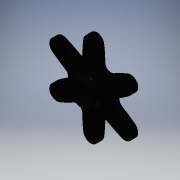
# Autodesk Inventor part: Sevo arm TowerPro SG-5010
Saved by Autodesk Inventor 2019 (Build 230136000, 136)
## iProperties
Created: 2015-05-13
Part Number: Sevo arm TowerPro SG-5010
Material: Ogólny
Document SubType Name: Modeling
Designer: Chaczyk
Density: 1 g/cm^3
Appearance: Domyślna
Author: Chaczyk
Autodesk Inventor part; units mm, degrees
ref_plane "YZ Plane" through (0, 0, 0) normal (1, 0, 0) x (0, 1, 0)
ref_plane "XZ Plane" through (0, 0, 0) normal (0, 1, 0) x (-1, 0, 0)
ref_plane "XY Plane" through (0, 0, 0) normal (0, 0, 1) x (1, 0, 0)
sketch "Szkic1" plane through (0, 0, 0) normal (0, 1, 0) x (-1, 0, 0)
  circle A0 centre (0, 0) radius 3.5
  line L0 (0, 0) -> (2.5, 0)
  line L1 (2.5, 0) -> (-2.5, 0)
  arc A1 (2.5, 13.012) -> (0, 15.5) centre (-0.142, 12.8573) ccw
  arc A2 (2.8239, 8.1091) -> (2.5, 13.012) centre (-52.6667, 6.905) ccw
  arc A3 (0, 15.5) -> (-2.5, 13.012) centre (0.142, 12.8573) ccw
  arc A4 (-2.5, 13.012) -> (-2.8239, 8.1091) centre (52.6667, 6.905) ccw
  circle A5 centre (0, 13.25) radius 0.5
  line L2 (3.8856, 6.386) -> (4.1618, 6.2393)
  arc A6 (2.8239, 8.1091) -> (3.8856, 6.386) centre (4.8235, 8.1525) ccw
  line L3 (-3.8856, 6.386) -> (-4.1618, 6.2393)
  arc A7 (-3.8856, 6.386) -> (-2.8239, 8.1091) centre (-4.8235, 8.1525) ccw
  line L4 (-4.1618, 6.2393) -> (4.1618, 6.2393)
  line L5 (0, 0) -> (0, 7.5)
  circle A8 centre (0, 7.5) radius 0.5
  line L6 (0, 13.25) -> (0, 7.5)
  circle A9 centre (0, 10.375) radius 0.5
  point P0 (2.837, 6.9427)
  point P1 (-2.837, 6.9427)
  dimension "d0" = 7
  dimension "d4" = 2.5
  dimension "d5" = 5
  dimension "d6" = 1
  dimension "d8" = 1.5
  dimension "d9" = 2
  dimension "d10" = 1.5
  dimension "d11" = 2
  dimension "d15" = 7.5
  dimension "d16" = 1
  dimension "d17" = 1
  constraints: 14 end point, 14 point on circle, 10 centre point, 4 tangent, 3 coincident, 3 point on line, 2 horizontal, 1 collinear, 1 midpoint, 1 vertical
  measures "d0" diameter of A0
  measures "d4" distance of L0.start L0.end
  measures "d5" distance of L0.end L1.end
  measures "d6" diameter of A5
  measures "d8" distance of point (2.837, 6.943) L2.end
  measures "d9" radius of A6
  measures "d10" distance of point (-2.837, 6.943) L3.end
  measures "d11" radius of A7
  measures "d15" distance of L0.start L5.end
  measures "d16" diameter of A8
  measures "d17" diameter of A9
sketch "Szkic2" plane through (0, 0, 0) normal (0, 1, 0) x (-1, 0, 0)
  circle A0 centre (0, 0) radius 7.5
  dimension "d12" = 15
  constraints: 1 centre point, 1 coincident
  measures "d12" diameter of A0
extrude "Wyciągnięcie proste1" add sketch "Szkic2" along normal blind 2
extrude "Wyciągnięcie proste2" add sketch "Szkic1" along normal blind 2 contours A2 A6 L2 L4 L3 A7 A4 A3 A1
pattern_circular "Szyk kołowy1" count 6 over 360 about axis through (0, 2, 0) along (0, 1, 0) of "Wyciągnięcie proste2"
sketch "Szkic3" plane through (0, 2, 0) normal (0, 1, 0) x (1, 0, 0)
  arc A0 (-0.4997, -7.4833) -> (0.4997, -7.4833) centre (0, 0) ccw projected
  circle A1 centre (0, -7.5) radius 0.5
  dimension "d23" = 1
  constraints: 1 centre point, 1 point on circle
  measures "d23" diameter of A1
extrude "Wyciągnięcie proste3" cut sketch "Szkic3" against normal blind 2
pattern_circular "Szyk kołowy2" count 6 over 360 about axis through (0, 2, 0) along (0, 1, 0) of "Wyciągnięcie proste3"
sketch "Szkic4" plane through (0, 2, 0) normal (0, 1, 0) x (1, 0, 0)
  circle A0 centre (0, 0) radius 3.5
  circle A1 centre (0, 0) radius 3.25
  dimension "d29" = 7
  dimension "d30" = 6.5
  constraints: 2 centre point, 2 coincident
  measures "d29" diameter of A0
  measures "d30" diameter of A1
extrude "Wyciągnięcie proste4" add sketch "Szkic4" along normal blind 0.5
sketch "Szkic5" plane through (0, 2, 0) normal (0, 1, 0) x (1, 0, 0)
  circle A0 centre (0, 0) radius 2
  dimension "d33" = 4
  constraints: 1 centre point, 1 coincident
  measures "d33" diameter of A0
extrude "Wyciągnięcie proste5" cut sketch "Szkic5" against normal blind 2
sketch "Szkic6" plane through (0, 0, 0) normal (0, -1, 0) x (1, 0, 0)
  circle A0 centre (0, 0) radius 4
  circle A1 centre (0, 0) radius 3.5
  dimension "d36" = 8
  dimension "d37" = 7
  constraints: 2 centre point, 2 coincident
  measures "d36" diameter of A0
  measures "d37" diameter of A1
extrude "Wyciągnięcie proste6" add sketch "Szkic6" along normal blind 3
fillet "Zaokrąglenie1" radius 2 1 edges at (-4, 0, 0)
fillet "Zaokrąglenie2" radius 0.25 1 edges at (-4, -3, 0)
fillet "Zaokrąglenie3" radius 0.25 1 edges at (-3.5, 2, 0)
sketch "Sketch7" plane through (0, 2, 0) normal (0, 1, 0) x (1, 0, 0)
  circle A0 centre (-6.4952, -3.75) radius 0.5 projected
  circle A1 centre (-6.4952, 3.75) radius 0.5 projected
  circle A2 centre (0, 7.5) radius 0.5 projected
  circle A3 centre (6.4952, 3.75) radius 0.5 projected
  circle A4 centre (6.4952, -3.75) radius 0.5 projected
  circle A5 centre (0, -7.5) radius 0.5 projected
  circle A6 centre (-11.4748, 6.625) radius 0.5 projected
  circle A7 centre (-8.985, 5.1875) radius 0.5 projected
  arc A8 (-5.6107, 6.5001) -> (-3.9339, 6.3855) centre (-4.6485, 8.2535) ccw projected
  arc A9 (-5.6107, 6.5001) -> (-10.0187, 8.6711) centre (-32.3132, -42.1582) ccw projected
  arc A10 (-10.0187, 8.6711) -> (-13.4234, 7.75) centre (-11.2058, 6.3057) ccw projected
  arc A11 (-13.4234, 7.75) -> (-12.5187, 4.3409) centre (-11.0638, 6.5516) ccw projected
  arc A12 (-12.5187, 4.3409) -> (-8.4346, 1.6089) centre (20.3535, 49.0631) ccw projected
  arc A13 (-7.4969, 0.2141) -> (-8.4346, 1.6089) centre (-9.472, -0.101) ccw projected
  arc A14 (-7.4969, 0.2141) -> (-7.4969, -0.2141) centre (0, 0) ccw projected
  arc A15 (-8.4346, -1.6089) -> (-7.4969, -0.2141) centre (-9.472, 0.101) ccw projected
  arc A16 (-8.4346, -1.6089) -> (-12.5187, -4.3409) centre (20.3535, -49.0631) ccw projected
  arc A17 (-12.5187, -4.3409) -> (-13.4234, -7.75) centre (-11.0638, -6.5516) ccw projected
  arc A18 (-13.4234, -7.75) -> (-10.0187, -8.6711) centre (-11.2058, -6.3057) ccw projected
  arc A19 (-10.0187, -8.6711) -> (-5.6107, -6.5001) centre (-32.3132, 42.1582) ccw projected
  arc A20 (-3.9339, -6.3855) -> (-5.6107, -6.5001) centre (-4.6485, -8.2535) ccw projected
  arc A21 (-3.9339, -6.3855) -> (-3.5631, -6.5996) centre (0, 0) ccw projected
  arc A22 (-2.8239, -8.1091) -> (-3.5631, -6.5996) centre (-4.8235, -8.1525) ccw projected
  arc A23 (-2.8239, -8.1091) -> (-2.5, -13.012) centre (52.6667, -6.905) ccw projected
  arc A24 (-2.5, -13.012) -> (0, -15.5) centre (0.142, -12.8573) ccw projected
  arc A25 (0, -15.5) -> (2.5, -13.012) centre (-0.142, -12.8573) ccw projected
  arc A26 (2.5, -13.012) -> (2.8239, -8.1091) centre (-52.6667, -6.905) ccw projected
  arc A27 (3.5631, -6.5996) -> (2.8239, -8.1091) centre (4.8235, -8.1525) ccw projected
  arc A28 (3.5631, -6.5996) -> (3.9339, -6.3855) centre (0, 0) ccw projected
  arc A29 (5.6107, -6.5001) -> (3.9339, -6.3855) centre (4.6485, -8.2535) ccw projected
  arc A30 (5.6107, -6.5001) -> (10.0187, -8.6711) centre (32.3132, 42.1582) ccw projected
  arc A31 (10.0187, -8.6711) -> (13.4234, -7.75) centre (11.2058, -6.3057) ccw projected
  arc A32 (13.4234, -7.75) -> (12.5187, -4.3409) centre (11.0638, -6.5516) ccw projected
  arc A33 (12.5187, -4.3409) -> (8.4346, -1.6089) centre (-20.3535, -49.0631) ccw projected
  arc A34 (7.4969, -0.2141) -> (8.4346, -1.6089) centre (9.472, 0.101) ccw projected
  arc A35 (7.4969, -0.2141) -> (7.4969, 0.2141) centre (0, 0) ccw projected
  arc A36 (8.4346, 1.6089) -> (7.4969, 0.2141) centre (9.472, -0.101) ccw projected
  arc A37 (8.4346, 1.6089) -> (12.5187, 4.3409) centre (-20.3535, 49.0631) ccw projected
  arc A38 (12.5187, 4.3409) -> (13.4234, 7.75) centre (11.0638, 6.5516) ccw projected
  arc A39 (13.4234, 7.75) -> (10.0187, 8.6711) centre (11.2058, 6.3057) ccw projected
  arc A40 (10.0187, 8.6711) -> (5.6107, 6.5001) centre (32.3132, -42.1582) ccw projected
  arc A41 (3.9339, 6.3855) -> (5.6107, 6.5001) centre (4.6485, 8.2535) ccw projected
  arc A42 (3.9339, 6.3855) -> (3.5631, 6.5996) centre (0, 0) ccw projected
  arc A43 (2.8239, 8.1091) -> (3.5631, 6.5996) centre (4.8235, 8.1525) ccw projected
  arc A44 (2.8239, 8.1091) -> (2.5, 13.012) centre (-52.6667, 6.905) ccw projected
  arc A45 (2.5, 13.012) -> (0, 15.5) centre (-0.142, 12.8573) ccw projected
  arc A46 (0, 15.5) -> (-2.5, 13.012) centre (0.142, 12.8573) ccw projected
  arc A47 (-2.5, 13.012) -> (-2.8239, 8.1091) centre (52.6667, 6.905) ccw projected
  arc A48 (-3.5631, 6.5996) -> (-2.8239, 8.1091) centre (-4.8235, 8.1525) ccw projected
  arc A49 (-3.5631, 6.5996) -> (-3.9339, 6.3855) centre (0, 0) ccw projected
  circle A50 centre (0, 13.25) radius 0.5 projected
  circle A51 centre (0, 10.375) radius 0.5 projected
  circle A52 centre (-8.985, -5.1875) radius 0.5 projected
  circle A53 centre (-11.4748, -6.625) radius 0.5 projected
  circle A54 centre (11.4748, 6.625) radius 0.5 projected
  circle A55 centre (8.985, 5.1875) radius 0.5 projected
  circle A56 centre (8.985, -5.1875) radius 0.5 projected
  circle A57 centre (11.4748, -6.625) radius 0.5 projected
  circle A58 centre (0, -13.25) radius 0.5 projected
  circle A59 centre (0, -10.375) radius 0.5 projected
  circle A60 centre (0, 0) radius 3.75 projected
  arc A61 (10.0187, -8.6711) -> (13.4234, -7.75) centre (11.2058, -6.3057) ccw projected
  arc A62 (0, -15.5) -> (2.5, -13.012) centre (-0.142, -12.8573) ccw projected
